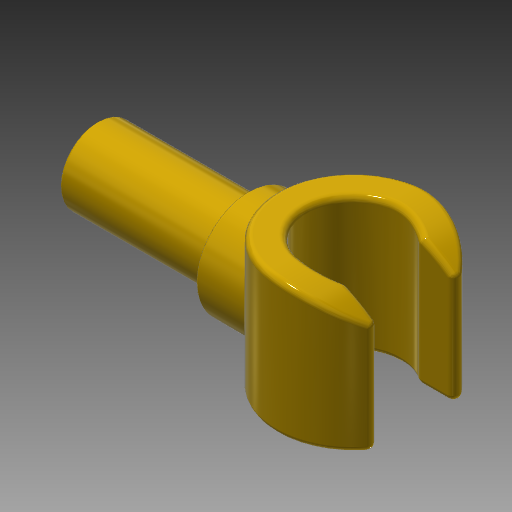
# Autodesk Inventor part: Mano Lego
Saved by Autodesk Inventor 2017 (Build 210142000, 142)
## iProperties
Created: 2017-06-23
Part Number: Mano Lego
Material: Plástico ABS
Document SubType Name: Modeling
Designer: H. Valenzuela B.
Density: 1.06 g/cm^3
Appearance: Suave - Blanco
Author: H. Valenzuela B.
Autodesk Inventor part; units mm, degrees
ref_plane "YZ Plane" through (0, 0, 0) normal (1, 0, 0) x (0, 1, 0)
ref_plane "XZ Plane" through (0, 0, 0) normal (0, 1, 0) x (-1, 0, 0)
ref_plane "XY Plane" through (0, 0, 0) normal (0, 0, 1) x (1, 0, 0)
sketch "Boceto1" plane through (0, 0, 0) normal (0, 0, 1) x (1, 0, 0)
  line L0 (-1.4, 0) -> (8.4, 0) construction
  line L1 (0, -0.35) -> (0, 2.1) construction
  line L2 (0, 0) -> (5, 0)
  line L3 (5, 0) -> (5, 1.25)
  line L4 (5, 1.25) -> (0, 1.25)
  line L5 (0, 1.25) -> (0, 0)
  line L6 (5, 0) -> (7, 0)
  line L7 (7, 0) -> (7, 1.75)
  line L8 (7, 1.75) -> (5, 1.75)
  line L9 (5, 1.75) -> (5, 0)
  dimension "d0" = 2.5
  dimension "d1" = 3.5
  dimension "d2" = 5
  dimension "d3" = 2
  constraints: 16 end point, 4 parallel, 2 horizontal, 2 perpendicular
  measures "d0" diameter of L4 L0
  measures "d1" diameter of L8 L0
  measures "d2" distance of L3.end L4.end
  measures "d3" distance of L7.end L8.end
revolve "Revolución1" add sketch "Boceto1" angle 360 about axis through (0, 0, 0) along (1, 0, 0)
sketch "Boceto2" plane through (0, 0, 0) normal (0, 1, 0) x (-1, 0, 0)
  circle A0 centre (-8.5, 0) radius 1.55
  line L0 (2.21, 0) -> (-13.26, 0) construction
  circle A1 centre (-8.5, 0) radius 2.55
  point P0 (0, 0)
  dimension "d5" = 3.1
  dimension "d6" = 5.1
  dimension "d7" = 8.5
  constraints: 2 centre point, 1 coincident, 1 point on line
  measures "d5" diameter of A0
  measures "d6" diameter of A1
  measures "d7" distance of A0.centre point (0, 0)
extrude "Extrusión1" add sketch "Boceto2" along normal mid plane 4.5
sketch "Boceto3" plane through (8.5, 2.25, 0) normal (0, 1, 0) x (1, 0, 0)
  circle A0 centre (0, 0) radius 1.55 projected
  line L0 (4.5081, -1.25) -> (0.4857, -1.25)
  line L1 (0.4857, -1.25) -> (0.4857, 1.25)
  line L2 (0.4857, 1.25) -> (4.5081, 1.25)
  line L3 (4.5081, 1.25) -> (4.5081, -1.25)
  line L4 (4.5081, -1.25) -> (0.4857, 1.25) construction
  line L5 (0.4857, -1.25) -> (4.5081, 1.25) construction
  line L6 (7.1097, 0) -> (-11.1016, 0) construction
  point P0 (-8.5, 0)
  point P1 (2.4969, 0)
  point P2 (2.4969, 0)
  dimension "d10" = 2.5
  constraints: 12 end point, 3 midpoint, 2 parallel, 1 horizontal, 1 perpendicular, 1 point on line
  measures "d10" distance between parallel lines of L0 L2
extrude "Extrusión2" cut sketch "Boceto3" along normal through all both and the other way through all
sketch "Boceto4" plane through (0, 0, 0) normal (0, 0, 1) x (1, 0, 0)
  line L0 (10.7226, -2.25) -> (10.7226, 2.25) construction
  line L1 (10.7226, 2.25) -> (5.95, 2.25) construction
  line L2 (6.95, 2.25) -> (9.4165, 2.25) projected
  arc A0 (10.7226, 1.25) -> (8.1095, 2.25) centre (8.1095, -1.6641) ccw
  line L3 (8.1095, 2.25) -> (8.1095, 5.971)
  line L4 (8.1095, 5.971) -> (10.7226, 5.971)
  line L5 (10.7226, 5.971) -> (10.7226, 1.25)
  point P0 (0, 0)
  dimension "d13" = 1
  constraints: 6 end point, 2 point on circle, 2 point on line, 1 centre point, 1 collinear, 1 perpendicular, 1 tangent, 1 vertical
  measures "d13" distance from line of L1 L5.end
extrude "Extrusión3" cut sketch "Boceto4" along normal through all both and the other way through all
fillet "Empalme1" radius 0.2 16 edges at (5.95, -2.25, 0) (6.95, -2.25, 0) (5.95, 2.25, 0) (9.7575, 1.8862, 2.2184) (9.7578, 1.886, -2.2182) (6.95, 2.25, 0) (8.8168, 2.1856, 1.5173) (8.8168, 2.1856, -1.5173) (10.1075, 1.7016, 1.25) (10.1075, 1.7016, -1.25) (10.0696, -2.25, 1.25) (10.0696, -2.25, -1.25) (9.4165, -0.1123, -1.25) (9.4165, -0.1123, 1.25) (10.7226, -0.5, 1.25) (10.7226, -0.5, -1.25)
fillet "Empalme2" radius 0.1 1 edges at (5, -1.75, 0)
fillet "Empalme3" radius 0.1 4 edges at (6.3077, 1.1688, 1.3024) (6.3077, -1.1688, 1.3024) (6.3077, 1.1688, -1.3024) (6.3077, -1.1688, -1.3024)
fillet "Empalme4" radius 0.1 1 edges at (5, -1.25, 0)
fillet "Empalme5" radius 0.1 1 edges at (0, -1.25, 0)
